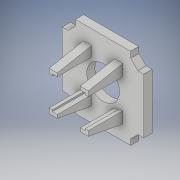
# Autodesk Inventor part: 20_Cube_Insert_Beamsplitter_v3
Saved by Autodesk Inventor 2019 (Build 230136000, 136)
## iProperties
Created: 2019-08-06
Part Number: 20_Cube_Insert_Beamsplitter_v3
Material: Generic
Document SubType Name: Modeling
Designer: marsikovabarbora
Density: 1 g/cm^3
Appearance: Default
Author: marsikovabarbora
Autodesk Inventor part; units mm, degrees
ref_plane "YZ Plane" through (0, 0, 0) normal (1, 0, 0) x (0, 1, 0)
ref_plane "XZ Plane" through (0, 0, 0) normal (0, 1, 0) x (-1, 0, 0)
ref_plane "XY Plane" through (0, 0, 0) normal (0, 0, 1) x (1, 0, 0)
sketch "Sketch1" plane through (0, 0, 0) normal (0, 0, 1) x (1, 0, 0)
  line L0 (-34.86, 0) -> (34.86, 0) construction
  line L1 (0, -34.86) -> (0, 34.86) construction
  line L2 (0, 0) -> (16.9726, 16.9726) construction
  line L3 (0, 0) -> (24.0028, 0) construction
  line L4 (0, 24.9) -> (16.8009, 24.9)
  line L5 (16.8009, 24.9) -> (16.8009, 21.2415)
  line L6 (16.8009, 21.2415) -> (19.0212, 19.0212)
  line L7 (24.9, 0) -> (24.9, 16.8009)
  line L8 (24.9, 16.8009) -> (21.2415, 16.8009)
  line L9 (21.2415, 16.8009) -> (19.0212, 19.0212)
  line L10 (0, -24.9) -> (16.8009, -24.9)
  line L11 (16.8009, -24.9) -> (16.8009, -21.2415)
  line L12 (16.8009, -21.2415) -> (19.0212, -19.0212)
  line L13 (24.9, 0) -> (24.9, -16.8009)
  line L14 (24.9, -16.8009) -> (21.2415, -16.8009)
  line L15 (21.2415, -16.8009) -> (19.0212, -19.0212)
  line L16 (0, 0) -> (-16.9726, 16.9726) construction
  line L17 (0, 0) -> (-24.0028, 0) construction
  line L18 (0, 24.9) -> (-16.8009, 24.9)
  line L19 (-16.8009, 24.9) -> (-16.8009, 21.2415)
  line L20 (-16.8009, 21.2415) -> (-19.0212, 19.0212)
  line L21 (-24.9, 0) -> (-24.9, 16.8009)
  line L22 (-24.9, 16.8009) -> (-21.2415, 16.8009)
  line L23 (-21.2415, 16.8009) -> (-19.0212, 19.0212)
  line L24 (0, -24.9) -> (-16.8009, -24.9)
  line L25 (-16.8009, -24.9) -> (-16.8009, -21.2415)
  line L26 (-16.8009, -21.2415) -> (-19.0212, -19.0212)
  line L27 (-21.2415, -16.8009) -> (-19.0212, -19.0212)
  line L28 (-24.9, -16.8009) -> (-21.2415, -16.8009)
  line L29 (-24.9, 0) -> (-24.9, -16.8009)
  circle A0 centre (0, 0) radius 10
  dimension "d17" = 45
  dimension "d18" = 24.9
  dimension "d20" = 3.14
  dimension "d21" = 26.9
  dimension "d22" = 20
  constraints: 56 end point, 22 symmetric about line, 3 point on line, 2 horizontal, 2 perpendicular, 1 centre point, 1 coincident, 1 equal length
  measures "d17" angle of L3 L2
  measures "d18" distance between parallel lines of L0 L4
  measures "d20" distance of L5.end L6.end
  measures "d21" distance from line of L2.start L6
  measures "d22" diameter of A0
extrude "Extrusion1" add sketch "Sketch1" along normal blind 5
sketch "Sketch2" plane through (0, 0, 5) normal (0, 0, 1) x (1, 0, 0)
  circle A0 centre (0, 0) radius 10 projected
  line L0 (16.8009, 24.9) -> (-16.8009, 24.9) projected
  line L1 (-16.8009, 24.9) -> (-16.8009, 21.2415) projected
  line L2 (-16.8009, 21.2415) -> (-21.2415, 16.8009) projected
  line L3 (-21.2415, 16.8009) -> (-24.9, 16.8009) projected
  line L4 (-24.9, 16.8009) -> (-24.9, -16.8009) projected
  line L5 (-24.9, -16.8009) -> (-21.2415, -16.8009) projected
  line L6 (-21.2415, -16.8009) -> (-16.8009, -21.2415) projected
  line L7 (-16.8009, -21.2415) -> (-16.8009, -24.9) projected
  line L8 (-16.8009, -24.9) -> (16.8009, -24.9) projected
  line L9 (16.8009, -24.9) -> (16.8009, -21.2415) projected
  line L10 (16.8009, -21.2415) -> (21.2415, -16.8009) projected
  line L11 (21.2415, -16.8009) -> (24.9, -16.8009) projected
  line L12 (24.9, -16.8009) -> (24.9, 16.8009) projected
  line L13 (24.9, 16.8009) -> (21.2415, 16.8009) projected
  line L14 (21.2415, 16.8009) -> (16.8009, 21.2415) projected
  line L15 (16.8009, 21.2415) -> (16.8009, 24.9) projected
  line L16 (0, -34.86) -> (0, 34.86) construction
  line L17 (-12, 12) -> (-7, 12)
  line L18 (-7, 12) -> (-7, 10)
  line L19 (-7, 10) -> (-12, 10)
  line L20 (-12, 10) -> (-12, 12)
  dimension "d27" = 2
  dimension "d28" = 5
  dimension "d29" = 12
  constraints: 8 end point, 2 parallel, 1 horizontal, 1 perpendicular, 1 tangent
  measures "d27" distance of L19.end L17.start
  measures "d28" distance of L17.start L17.end
  measures "d29" distance between parallel lines of L16 L20
extrude "Extrusion2" add sketch "Sketch2" along normal blind 21 contours L17 L18 L19 L20
sketch "Sketch4" plane through (-12, 10, 5) normal (-1, 0, 0) x (0, 0, 1)
  line L0 (0, 0) -> (0, 2) projected
  line L1 (0, 0) -> (21, 0) projected
  line L2 (21, 2) -> (21, 0) projected
  line L3 (0, 2) -> (21, 2) projected
  line L4 (0, 6.8009) -> (0, -26.8009) projected
  line L5 (0, 2) -> (21, 2) projected
  line L6 (21, 2) -> (0, 2)
  line L7 (0, 2) -> (0, 6)
  line L8 (0, -26.8009) -> (0, 6.8009) projected
  line L9 (0, 6) -> (21, 2)
  point P0 (-5, -10)
  dimension "d35" = 4
  constraints: 6 end point, 1 perpendicular, 1 point on line
  measures "d35" distance of L0.end L7.end
extrude "Extrusion4" add sketch "Sketch4" against normal up to surface (5 mm away) contours L4 L9 L3
sketch "Sketch5" plane through (-12, 10, 5) normal (0, -1, 0) x (1, 0, 0)
  line L0 (5, 21) -> (5, 0) projected
  line L1 (0, 0) -> (5, 0) projected
  line L2 (0, 21) -> (0, 0) projected
  line L3 (5, 21) -> (0, 21) projected
  line L4 (12, -10.2) -> (12, 26.2) construction
  line L5 (0, 21) -> (2, 21)
  line L6 (2, 21) -> (2, 0)
  line L7 (2, 0) -> (0, 0)
  line L8 (0, 0) -> (0, 21)
  point P0 (12, -5)
  dimension "d38" = 10
  constraints: 8 end point, 2 parallel, 1 horizontal, 1 perpendicular, 1 point on line
  measures "d38" distance between parallel lines of L4 L6
extrude "Extrusion5" add sketch "Sketch5" along normal blind 1 contours L6 L1 L2 L3
mirror "Mirror1" about plane through (0, 0, 0) normal (0, 1, 0) of "Extrusion2", "Extrusion4", "Extrusion5"
mirror "Mirror2" about plane through (0, 0, 0) normal (1, 0, 0) of "Extrusion2", "Extrusion4", "Mirror1", "Extrusion5"
sketch "Skizze6" plane through (0, 0, 5) normal (0, 0, 1) x (1, 0, 0)
  line L0 (12, -16) -> (7, -16) construction
  line L1 (7, -16) -> (7, -10) construction
  line L2 (7, -10) -> (10, -10) construction
  line L3 (10, -10) -> (10, -9) construction
  line L4 (10, -9) -> (12, -9) construction
  line L5 (12, -9) -> (12, -16) construction
  line L6 (7, 16) -> (12, 16) construction
  line L7 (12, 16) -> (12, 9) construction
  line L8 (12, 9) -> (10, 9) construction
  line L9 (10, 9) -> (10, 10) construction
  line L10 (10, 10) -> (7, 10) construction
  line L11 (7, 10) -> (7, 16) construction
  line L12 (-7, -16) -> (-12, -16) construction
  line L13 (-12, -16) -> (-12, -9) construction
  line L14 (-12, -9) -> (-10, -9) construction
  line L15 (-10, -9) -> (-10, -10) construction
  line L16 (-10, -10) -> (-7, -10) construction
  line L17 (-7, -10) -> (-7, -16) construction
  line L18 (-12, 9) -> (-12, 16) construction
  line L19 (-12, 16) -> (-7, 16) construction
  line L20 (-7, 16) -> (-7, 10) construction
  line L21 (-7, 10) -> (-10, 10) construction
  line L22 (-10, 10) -> (-10, 9) construction
  line L23 (-10, 9) -> (-12, 9) construction
  circle A0 centre (0, 0) radius 10 construction
  line L24 (16.8009, 24.9) -> (-16.8009, 24.9) construction
  line L25 (-16.8009, 24.9) -> (-16.8009, 21.2415) projected
  line L26 (-16.8009, 21.2415) -> (-21.2415, 16.8009) projected
  line L27 (-21.2415, 16.8009) -> (-24.9, 16.8009) projected
  line L28 (-24.9, 16.8009) -> (-24.9, -16.8009) construction
  line L29 (-24.9, -16.8009) -> (-21.2415, -16.8009) projected
  line L30 (-21.2415, -16.8009) -> (-16.8009, -21.2415) projected
  line L31 (-16.8009, -21.2415) -> (-16.8009, -24.9) projected
  line L32 (-16.8009, -24.9) -> (16.8009, -24.9) construction
  line L33 (16.8009, -24.9) -> (16.8009, -21.2415) projected
  line L34 (16.8009, -21.2415) -> (21.2415, -16.8009) projected
  line L35 (21.2415, -16.8009) -> (24.9, -16.8009) projected
  line L36 (24.9, -16.8009) -> (24.9, 16.8009) construction
  line L37 (24.9, 16.8009) -> (21.2415, 16.8009) projected
  line L38 (21.2415, 16.8009) -> (16.8009, 21.2415) projected
  line L39 (16.8009, 21.2415) -> (16.8009, 24.9) projected
  line L40 (-16.9009, 25) -> (16.9009, 25) construction
  line L41 (16.9009, 25) -> (16.9009, 21.2829)
  line L42 (16.9009, 21.2829) -> (21.2829, 16.9009)
  line L43 (21.2829, 16.9009) -> (25, 16.9009)
  line L44 (25, 16.9009) -> (25, -16.9009) construction
  line L45 (25, -16.9009) -> (21.2829, -16.9009)
  line L46 (21.2829, -16.9009) -> (16.9009, -21.2829)
  line L47 (16.9009, -21.2829) -> (16.9009, -25)
  line L48 (16.9009, -25) -> (-16.9009, -25) construction
  line L49 (-16.9009, -25) -> (-16.9009, -21.2829)
  line L50 (-16.9009, -21.2829) -> (-21.2829, -16.9009)
  line L51 (-21.2829, -16.9009) -> (-25, -16.9009)
  line L52 (-25, -16.9009) -> (-25, 16.9009) construction
  line L53 (-25, 16.9009) -> (-21.2829, 16.9009)
  line L54 (-21.2829, 16.9009) -> (-16.9009, 21.2829)
  line L55 (-16.9009, 21.2829) -> (-16.9009, 25)
  line L56 (-24.9, 16.8009) -> (-24.9, 16.9009)
  line L57 (-16.8009, 24.9) -> (-16.9009, 24.9)
  line L58 (16.8009, 24.9) -> (-16.8009, 24.9) projected
  line L59 (16.8009, 24.9) -> (16.9009, 24.9)
  line L60 (24.9, 16.8009) -> (24.9, 16.9009)
  line L61 (16.8009, -24.9) -> (16.9009, -24.9)
  line L62 (21.2415, -16.8009) -> (24.9, -16.8009) projected
  line L63 (24.9, -16.8009) -> (24.9, -16.9009)
  line L64 (-16.8009, -24.9) -> (-16.9009, -24.9)
  line L65 (-24.9, -16.8009) -> (-21.2415, -16.8009) projected
  line L66 (-24.9, -16.8009) -> (-24.9, -16.9009)
  dimension "d17" = 45
  dimension "d18" = 24.9
  dimension "d20" = 3.14
  dimension "d21" = 26.9
  dimension "d41" = 0.1
  constraints: 48 end point, 12 point on line, 3 perpendicular, 1 vertical, 15 other
  measures "d41" distance between parallel lines of L24 L40
extrude "IM_offset" add sketch "Skizze6" against normal up to surface (5 mm away)
body "Solid1"
